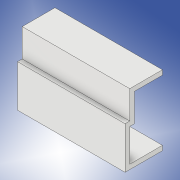
# Autodesk Inventor part: FA003
Saved by Autodesk Inventor 2017 SP1 (Build 210196100, 196)
## iProperties
Created: 2017-06-16
Part Number: FA003
Material: ABS Plastic
Document SubType Name: Modeling
Designer: Zach
Density: 1.06 g/cm^3
Appearance: CR White
Author: Zach
Autodesk Inventor part; units mm, degrees
ref_plane "YZ Plane" through (0, 0, 0) normal (1, 0, 0) x (0, 1, 0)
ref_plane "XZ Plane" through (0, 0, 0) normal (0, 1, 0) x (-1, 0, 0)
ref_plane "XY Plane" through (0, 0, 0) normal (0, 0, 1) x (1, 0, 0)
sketch "Sketch1" plane through (0, 0, 0) normal (0, 0, 1) x (1, 0, 0)
  line L0 (0, 0) -> (115, 0)
  line L1 (115, 0) -> (115, 75)
  line L2 (115, 75) -> (0, 75)
  line L3 (0, 75) -> (0, 0)
  dimension "d0" = 115
  dimension "d1" = 75
  constraints: 8 end point, 2 parallel, 1 horizontal, 1 perpendicular
  measures "d0" distance of L2.end L1.end
  measures "d1" distance of L1.end L0.end
extrude "Extrusion1" add sketch "Sketch1" along normal blind 40
sketch "Sketch2" plane through (0, 0, 40) normal (0, 0, 1) x (1, 0, 0)
  line L0 (115, 75) -> (0, 75) projected
  line L1 (115, 0) -> (115, 75) projected
  line L2 (0, 75) -> (115, 75)
  line L3 (115, 75) -> (115, 45)
  line L4 (115, 45) -> (0, 45)
  line L5 (0, 45) -> (0, 75)
  point P0 (0, 0)
  dimension "d4" = 30
  constraints: 8 end point, 2 parallel, 1 horizontal, 1 perpendicular, 1 point on line
  measures "d4" distance of L2.end L3.end
extrude "Extrusion2" cut sketch "Sketch2" against normal blind 5
sketch "Sketch3" plane through (115, 0, 0) normal (1, 0, 0) x (0, 0, -1)
  line L0 (0, 75) -> (-35, 75) projected
  line L1 (-35, 75) -> (-35, 45) projected
  line L2 (-35, 45) -> (-40, 45) projected
  line L3 (-40, 0) -> (-40, 45) projected
  line L4 (0, 0) -> (-40, 0) projected
  line L5 (0, 70) -> (-30, 70)
  line L6 (-30, 70) -> (-30, 40)
  line L7 (-30, 40) -> (-35, 40)
  line L8 (-35, 40) -> (-35, 5)
  line L9 (-35, 5) -> (0, 5)
  line L10 (0, 5) -> (0, 70)
  line L11 (0, 0) -> (0, 75) projected
  dimension "d7" = 5
  constraints: 12 end point, 1 collinear, 4 other
  measures "d7" distance between parallel lines of L0 L5
extrude "Extrusion3" cut sketch "Sketch3" against normal through all contours L10 L9 L8 L7 L6 L5
body "Solid1"
